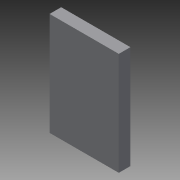
# Autodesk Inventor part: intocircuit 26Ah
Saved by Autodesk Inventor 2015 (Build 190159000, 159)
## iProperties
Created: 2014-09-20
Part Number: intocircuit 26Ah
Material: Generic
Document SubType Name: Modeling
Designer: ericd_000
Density: 1 g/cm^3
Appearance: Default
Author: ericd_000
Autodesk Inventor part; units mm, degrees
ref_plane "YZ Plane" through (0, 0, 0) normal (1, 0, 0) x (0, 1, 0)
ref_plane "XZ Plane" through (0, 0, 0) normal (0, 1, 0) x (-1, 0, 0)
ref_plane "XY Plane" through (0, 0, 0) normal (0, 0, 1) x (1, 0, 0)
sketch "Sketch1" plane through (0, 0, 0) normal (0, 1, 0) x (-1, 0, 0)
  line L0 (56.3133, 79.1104) -> (-68.6867, 79.1104)
  line L1 (-68.6867, 79.1104) -> (-68.6867, -106.8896)
  line L2 (-68.6867, -106.8896) -> (56.3133, -106.8896)
  line L3 (56.3133, -106.8896) -> (56.3133, 79.1104)
  point P0 (0, 0)
  dimension "d0" = 186
  dimension "d1" = 125
  constraints: 8 end point, 2 parallel, 1 horizontal, 1 perpendicular
  measures "d0" distance of L2.end L0.start
  measures "d1" distance of L0.start L0.end
extrude "Extrusion1" add sketch "Sketch1" along normal blind 21
body "Solid1"
